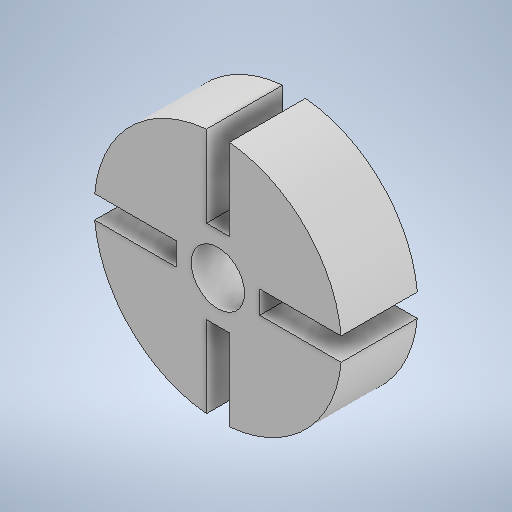
# Autodesk Inventor part: Rotor
Saved by Autodesk Inventor 2026.1 (Build 301233020, 233B)
## iProperties
Created: 2025-10-20
Part Number: Rotor
Material: Generic
Document SubType Name: Modeling
Designer: yo
Density: 1 g/cm^3
Appearance: Default
Author: yo
Autodesk Inventor part; units mm, degrees
ref_plane "YZ Plane" through (0, 0, 0) normal (1, 0, 0) x (0, 1, 0)
ref_plane "XZ Plane" through (0, 0, 0) normal (0, 1, 0) x (-1, 0, 0)
ref_plane "XY Plane" through (0, 0, 0) normal (0, 0, 1) x (1, 0, 0)
sketch "Sketch1" plane through (0, 0, 0) normal (0, 0, 1) x (1, 0, 0)
  circle A0 centre (0, 0) radius 16.25
  line L0 (0, 16.25) -> (0, -16.25) construction
  line L1 (-16.25, 0) -> (16.25, 0) construction
  line L2 (-1.5, 16.1806) -> (-1.5, 5.4806)
  line L3 (1.5, 16.1806) -> (1.5, 5.4806)
  line L4 (-1.5, 5.4806) -> (1.5, 5.4806)
  line L5 (-16.1806, 1.5) -> (-5.4806, 1.5)
  line L6 (-5.4806, -1.5) -> (-5.4806, 1.5)
  line L7 (-16.1806, -1.5) -> (-5.4806, -1.5)
  line L8 (-1.5, -16.1806) -> (-1.5, -5.4806)
  line L9 (1.5, -5.4806) -> (-1.5, -5.4806)
  line L10 (1.5, -16.1806) -> (1.5, -5.4806)
  line L11 (16.1806, -1.5) -> (5.4806, -1.5)
  line L12 (5.4806, 1.5) -> (5.4806, -1.5)
  line L13 (16.1806, 1.5) -> (5.4806, 1.5)
  circle A1 centre (0, 0) radius 3.5
  point P0 (0, 5.4806)
  point P1 (-5.4806, 0)
  point P2 (0, -5.4806)
  point P3 (5.4806, 0)
  dimension "d1" = 3
  dimension "d2" = 10.7
  dimension "d5" = 360
  dimension "d7" = 7
  dimension "d12" = 32.5
  constraints: 28 end point, 6 point on circle, 4 coincident, 3 midpoint, 3 vertical, 2 centre point, 2 perpendicular, 1 parallel, 1 vertical alignment, 33 other
  measures "d1" diameter of L2 L0
  measures "d2" distance of L2.start L2.end
  measures "d7" diameter of A1
  measures "d12" diameter of A0
extrude "Extrusion1" add sketch "Sketch1" along normal mid plane 10 contours L13 L12 L11 A0 L10 L9 L8 L7 L6 L5 L2 L4 L3
body "Solid1"
